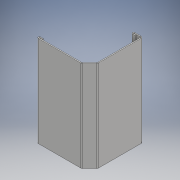
# Autodesk Inventor part: 4-5
Saved by Autodesk Inventor 2017 (Build 210142000, 142)
## iProperties
Part Number: 4-5
Material: 一般
Document SubType Name: 板金
Designer: Brian
Density: 1 g/cm^3
Sheet Metal Rule: 預設
Appearance: 預設
Author: Brian
Autodesk Inventor part; units mm, degrees
ref_plane "YZ Plane" through (0, 0, 0) normal (1, 0, 0) x (0, 1, 0)
ref_plane "XZ Plane" through (0, 0, 0) normal (0, 1, 0) x (-1, 0, 0)
ref_plane "XY Plane" through (0, 0, 0) normal (0, 0, 1) x (1, 0, 0)
sketch "草圖1" plane through (0, 0, 0) normal (0, 1, 0) x (-1, 0, 0)
  line L0 (0, 0) -> (-94, 0)
  line L1 (-94, 0) -> (-94, -192)
  line L2 (-94, -192) -> (0, -192)
  line L3 (0, -192) -> (0, 0)
  dimension "d0" = 192
  dimension "d1" = 94
  measures "d0" distance of L2.end L0.start
  measures "d1" distance of L0.start L0.end
extrude "平板1" add sketch "草圖1" along normal blind 2
sketch "草圖2" plane through (92.5858, 1.4142, -192) normal (0.7071068, -0.7071068, 0) x (0.7071068, 0.7071068, 0)
  line L0 (0, 192) -> (0, 0)
  line L1 (0, 0) -> (24.038, 0)
  line L2 (24.038, 0) -> (24.038, 192)
  line L3 (24.038, 192) -> (0, 192)
  constraints: 6 end point, 1 horizontal, 1 perpendicular, 1 vertical
edge flange "凸緣1" height 24.038 angle 45 thickness 2 bend radius 2 thickness toward (0.7071068, -0.7071068, 0) relief tear relief width 2 relief depth 1 edges at (94, 2, -96) wall of the first edge with corners at (92.5858, 1.4142, 0) (92.5858, 1.4142, -192) (109.5832, 18.4116, -192) (109.5832, 18.4116, 0)
bend "折彎1"
corner "轉角1"
sketch "草圖3" plane through (108.9974, 16.9974, -192) normal (1, 0, 0) x (0, 1, 0)
  line L0 (0, 192) -> (0, 0)
  line L1 (0, 0) -> (95.6, 0)
  line L2 (95.6, 0) -> (95.6, 192)
  line L3 (95.6, 192) -> (0, 192)
  constraints: 6 end point, 1 horizontal, 1 perpendicular, 1 vertical
edge flange "凸緣2" height 95.6 angle 45 thickness 2 bend radius 2 thickness toward (1, 0, 0) relief tear relief width 2 relief depth 1 edges at (109.5832, 18.4116, -96) wall of the first edge with corners at (108.9974, 16.9974, 0) (108.9974, 16.9974, -192) (108.9974, 112.5974, -192) (108.9974, 112.5974, 0)
bend "折彎2"
corner "轉角2"
sketch "草圖4" plane through (110.9974, 110.5974, -192) normal (0, 1, 0) x (-1, 0, 0)
  line L0 (0, 192) -> (0, 0)
  line L1 (0, 0) -> (19.5, 0)
  line L2 (19.5, 0) -> (19.5, 192)
  line L3 (19.5, 192) -> (0, 192)
  constraints: 6 end point, 1 horizontal, 1 perpendicular, 1 vertical
edge flange "凸緣3" height 19.5 angle 90 thickness 2 bend radius 2 thickness toward (0, 1, 0) relief tear relief width 2 relief depth 1 edges at (108.9974, 112.5974, -96) wall of the first edge with corners at (110.9974, 110.5974, 0) (110.9974, 110.5974, -192) (91.4974, 110.5974, -192) (91.4974, 110.5974, 0)
bend "折彎3"
corner "轉角3"
sketch "草圖5" plane through (93.9974, 110.5974, 0) normal (0, 0, 1) x (1, 0, 0)
  line L0 (0, 2) -> (0, 0)
  arc A0 (0, 0) -> (0, -1) centre (0, -0.5) ccw
  line L1 (0, -1) -> (6, -1)
  line L2 (6, -1) -> (6, -3)
  line L3 (6, -3) -> (0, -3)
  arc A1 (0, 2) -> (0, -3) centre (0, -0.5) ccw
  constraints: 8 end point, 4 point on circle
hem "折邊1" sketch "草圖5" thickness 2 along (0, 0, -1) edges at (91.4974, 110.5974, -96)
sketch "草圖6" plane through (2.5, 2, -192) normal (0, 0, -1) x (-1, 0, 0)
  line L0 (0, -2) -> (0, 0)
  arc A0 (0, 0) -> (0, 1) centre (0, 0.5) ccw
  line L1 (0, 1) -> (-6, 1)
  line L2 (-6, 1) -> (-6, 3)
  line L3 (-6, 3) -> (0, 3)
  arc A1 (0, -2) -> (0, 3) centre (0, 0.5) ccw
  constraints: 8 end point, 4 point on circle
hem "折邊2" sketch "草圖6" thickness 2 along (0, 0, 1) edges at (0, 2, -96)
equation "\"d33\" = 折彎離隙寬度"
equation "\"d34\" = 折彎離隙深度"
equation "\"d35\" = 最小剩餘"
equation "\"d36\" = 折彎半徑"
equation "\"d38\" = 0.5 * 厚度"
equation "\"d39\" = 0.5 * d38"
equation "\"d40\" = 折彎離隙寬度"
equation "\"d41\" = 折彎離隙深度"
equation "\"d42\" = 最小剩餘"
equation "\"d43\" = 折彎半徑"
equation "\"d45\" = 0.5 * 厚度"
equation "\"d46\" = 0.5 * d45"
equation "\"d3\" = 折彎離隙寬度"
equation "\"d4\" = 折彎離隙深度"
equation "\"d5\" = 最小剩餘"
equation "\"d6\" = 折彎半徑"
equation "\"d9\" = 折彎半徑"
equation "\"d10\" = 轉角離隙大小"
equation "\"d11\" = 間隙大小"
equation "\"d12\" = Jacobi半徑大小"
equation "\"d13\" = 折彎離隙寬度"
equation "\"d14\" = 折彎離隙深度"
equation "\"d15\" = 最小剩餘"
equation "\"d16\" = 折彎半徑"
equation "\"d19\" = 折彎半徑"
equation "\"d20\" = 轉角離隙大小"
equation "\"d21\" = 間隙大小"
equation "\"d22\" = Jacobi半徑大小"
equation "\"d23\" = 折彎離隙寬度"
equation "\"d24\" = 折彎離隙深度"
equation "\"d25\" = 最小剩餘"
equation "\"d26\" = 折彎半徑"
equation "\"d29\" = 折彎半徑"
equation "\"d30\" = 轉角離隙大小"
equation "\"d31\" = 間隙大小"
equation "\"d32\" = Jacobi半徑大小"
equation "\"折彎半徑\" = 厚度"
equation "\"折彎離隙寬度\" = 厚度"
equation "\"折彎離隙深度\" = 0.5 * 厚度"
equation "\"轉角離隙大小\" = 4 * 厚度"
equation "\"最小剩餘\" = 2 * 厚度"
equation "\"轉移半徑\" = 折彎半徑"
equation "\"Jacobi半徑大小\" = 厚度"
equation "\"間隙大小\" = 厚度"
equation "\"d2\" = 折彎半徑"
equation "\"厚度\" = 2"
